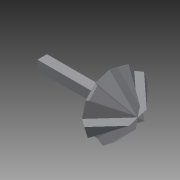
# Autodesk Inventor part: RotateGear
Saved by Autodesk Inventor 2015 (Build 190159000, 159)
## iProperties
Created: 2015-06-17
Part Number: RotateGear
Material: Generic
Document SubType Name: Modeling
Designer: david_000
Density: 1 g/cm^3
Appearance: Default
Author: david_000
Autodesk Inventor part; units mm, degrees
ref_plane "YZ Plane" through (0, 0, 0) normal (1, 0, 0) x (0, 1, 0)
ref_plane "XZ Plane" through (0, 0, 0) normal (0, 1, 0) x (-1, 0, 0)
ref_plane "XY Plane" through (0, 0, 0) normal (0, 0, 1) x (1, 0, 0)
sketch "Sketch6" plane through (0, 0, 0) normal (1, 0, 0) x (0, 1, 0)
  line L0 (5.2569, 0.1572) -> (4.6312, -2.4922)
  line L1 (4.6312, -2.4922) -> (2.7646, -4.4739)
  line L2 (2.7646, -4.4739) -> (0.1572, -5.2569)
  line L3 (0.1572, -5.2569) -> (-2.4922, -4.6312)
  line L4 (-2.4922, -4.6312) -> (-4.4739, -2.7646)
  line L5 (-4.4739, -2.7646) -> (-5.2569, -0.1572)
  line L6 (-5.2569, -0.1572) -> (-4.6312, 2.4922)
  line L7 (-4.6312, 2.4922) -> (-2.7646, 4.4739)
  line L8 (-2.7646, 4.4739) -> (-0.1572, 5.2569)
  line L9 (-0.1572, 5.2569) -> (2.4922, 4.6312)
  line L10 (2.4922, 4.6312) -> (4.4739, 2.7646)
  line L11 (4.4739, 2.7646) -> (5.2569, 0.1572)
  point P0 (0, 0)
  point P1 (0, 0)
  dimension "d27" = 5.08
  constraints: 24 end point, 1 coincident, 25 other
  measures "d27" distance from line of point (0, 0) L8
extrude "Extrusion2" add sketch "Sketch6" along normal blind 6.096 draft -45
sketch "Sketch7" plane through (0, 2.4922, 4.6312) normal (0.7071068, 0.484827, 0.5147259) x (0, 0.7279324, -0.6856489)
  line L0 (0, 0) -> (2.7224, 0)
  line L1 (0, 0) -> (2.7224, 0) projected
  line L2 (2.7224, 0) -> (1.3511, -7.2372)
  line L3 (2.7224, 0) -> (1.3612, -7.1842) projected
  line L4 (1.3511, -7.2372) -> (0, 0)
  point P0 (1.3612, -3.5921)
  dimension "d38" = 0
  dimension "d30" = 7.366
  constraints: 6 end point, 2 collinear
  measures "d30" distance of L0.end L2.end
extrude "Extrusion3" add sketch "Sketch7" along normal blind 1.27 draft -10
sketch "Sketch8" plane through (0, 0, 0) normal (-1, 0, 0) x (0, 0, 1)
  line L0 (-0.889, -0.889) -> (0.889, -0.889)
  line L1 (0.889, -0.889) -> (0.889, 0.889)
  line L2 (0.889, 0.889) -> (-0.889, 0.889)
  line L3 (-0.889, 0.889) -> (-0.889, -0.889)
  line L4 (-0.889, -0.889) -> (0.889, 0.889) construction
  line L5 (0.889, -0.889) -> (-0.889, 0.889) construction
  point P0 (0, 0)
  dimension "d33" = 1.778
  dimension "d34" = 1.778
  constraints: 12 end point, 2 midpoint, 2 parallel, 1 horizontal, 1 perpendicular
  measures "d33" distance of L2.end L1.end
  measures "d34" distance of L1.end L0.end
extrude "Extrusion4" add sketch "Sketch8" along normal blind 12.7
sketch "Sketch9" plane through (-12.7, 0, 0) normal (-1, 0, 0) x (0, 0, 1)
  circle A0 centre (0, 0) radius 0.0758
  point P0 (0, 0)
  constraints: 2 coincident, 1 centre point
extrude "Extrusion5" add sketch "Sketch9" along normal blind 0.0254
pattern_circular "Circular Pattern1" count 6 over 360 about axis through (-12.7, 0, 0) along (-1, 0, 0) of "Extrusion3"
body "Solid2"
